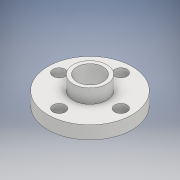
# Autodesk Inventor part: Piping_Flange_1in
Saved by Autodesk Inventor 2018 (Build 220112000, 112)
## iProperties
Created: 2018-10-12
Part Number: Piping_Flange_1in
Material: PVC-Piping
Document SubType Name: Modeling
Designer: Bradley
Density: 1.4 g/cm^3
Appearance: Smooth - White
Author: Bradley
Autodesk Inventor part; units mm, degrees
ref_plane "YZ Plane" through (0, 0, 0) normal (1, 0, 0) x (0, 1, 0)
ref_plane "XZ Plane" through (0, 0, 0) normal (0, 1, 0) x (-1, 0, 0)
ref_plane "XY Plane" through (0, 0, 0) normal (0, 0, 1) x (1, 0, 0)
sketch "Sketch1" plane through (0, 0, 0) normal (0, 1, 0) x (-1, 0, 0)
  line L0 (-12.954, -17.4625) -> (-12.954, -14.2875)
  line L1 (-12.954, -14.2875) -> (-16.8275, -14.2875)
  line L2 (-16.8275, -14.2875) -> (-16.8275, 17.4625)
  line L3 (-16.8275, 17.4625) -> (-21.59, 17.4625)
  line L4 (-21.59, 17.4625) -> (-21.59, -0.6985)
  line L5 (-21.59, -0.6985) -> (-53.975, -0.6985)
  line L6 (-53.975, -0.6985) -> (-53.975, -17.4625)
  line L7 (-53.975, -17.4625) -> (-12.954, -17.4625)
  line L8 (0, -17.4625) -> (0, 17.4625)
  point P0 (0, 0)
  point P1 (0, 0)
  dimension "d0" = 3.175
  dimension "d1" = 34.925
  dimension "d2" = 33.655
  dimension "d3" = 107.95
  dimension "d4" = 43.18
  dimension "d5" = 25.908
  dimension "d6" = 16.764
  constraints: 18 end point, 8 perpendicular, 2 point on line, 1 coincident, 1 midpoint, 1 vertical
  measures "d0" distance between parallel lines of L7 L1
  measures "d1" distance between parallel lines of L7 L3
  measures "d2" diameter of L2 L8
  measures "d3" diameter of L6 L8
  measures "d4" diameter of L4 L8
  measures "d5" diameter of L0 L8
  measures "d6" distance between parallel lines of L7 L5
revolve "Revolution1" add sketch "Sketch1" angle 360 about axis through (0, 0, -17.4625) along (0, 0, 1)
sketch "Sketch2" plane through (0, 0, -0.6985) normal (0, 0, 1) x (1, 0, 0)
  point P0 (0, 0)
  point P1 (0, -39.6875)
  point P2 (39.6875, 0)
  point P3 (0, 39.6875)
  point P4 (-39.6875, 0)
  dimension "d10" = 360
  dimension "d12" = 79.375
  constraints: 1 vertical alignment, 5 other
  measures "d12" distance of point (0, 39.688) point (0, -39.688)
hole "Hole1" at (0, -39.6875, -0.6985) at (39.6875, 0, -0.6985) at (0, 39.6875, -0.6985) at (-39.6875, 0, -0.6985) direction (0, 0, -1) diameter 15.875 end through all
body "Solid1"
